Autodesk Fusion 360 part; units mm, degrees
note: some values were not read from the file. Set by a fixed rule: which face or edge a step refers to.
(part 2 of 2)
sketch "Sketch1 (6)" plane through (0, -1, 0) normal (0, -1, 0) x (1, 0, 0) in component "RightBoardHolder"
  circle A0 centre (157, 114) radius 1.35
  circle A1 centre (157, 114) radius 4
  line L0 (157, 118) -> (103, 118)
  line L1 (103, 118) -> (103, 54)
  arc A2 (103, 54) -> (161, 114) centre (100.9655, 114) ccw
  line L2 (103, 118) -> (75, 118)
  line L3 (75, 118) -> (103, 118)
  line L4 (103, 118) -> (103, 54)
  line L5 (103, 54) -> (75, 54)
  line L6 (75, 54) -> (75, 118)
  line L7 (75, 54) -> (95, 54)
  line L8 (95, 54) -> (75, 54)
  line L9 (75, 54) -> (75, 88)
  line L10 (75, 88) -> (95, 88)
  line L11 (95, 88) -> (95, 54)
  dimension "d287" = 54
  dimension "d288" = 64
  dimension "d304" = 28
  dimension "d363" = 20
  dimension "d364" = 34
  constraint coincident A1 L0.start
  constraint horizontal L0
  constraint perpendicular L0 L1
  constraint tangent A1 A2
  constraint coincident A1 A2.end
  constraint perpendicular L1 L2
  constraint horizontal L3
  constraint vertical L4
  constraint horizontal L5
  constraint vertical L6
  constraint perpendicular L6 L7
  constraint horizontal L8
  constraint vertical L9
  constraint horizontal L10
  constraint vertical L11
  measures "d287" distance of L0.start L0.end
  measures "d288" distance of L0.end L1.end
  measures "d304" distance of L0.end L2.end
  measures "d363" distance of L5.end L7.end
  measures "d364" distance of L7.end L10.end
extrude "Extrude1'''''" add sketch "Sketch1 (6)" along normal blind 2 separate body contours A1 | A1 L0 L1 A2 L4 | L1 L2 L3 L4 L5 L6 L10 L11 makes body 8 in component "RightBoardHolder"
sketch "Sketch2 (6)" plane through (0, -1, 0) normal (0, 1, 0) x (-1, 0, 0) in component "RightBoardHolder"
  circle A0 centre (-157, 114) radius 1.35
  arc A1 (-161, 114) -> (-103, 54) centre (-100.9655, 114) ccw
  line L0 (-75, 118) -> (-157, 118)
  arc A2 (-157, 118) -> (-161, 114) centre (-157, 114) ccw
  line L1 (-157, 114) -> (-127, 114)
  line L2 (-127, 114) -> (-95, 114)
  line L3 (-95, 114) -> (-95, 67)
  line L4 (-95, 67) -> (-127, 67)
  line L5 (-127, 67) -> (-127, 114)
  line L6 (-103, 54) -> (-95, 54)
  line L7 (-75, 88) -> (-75, 118)
  line L8 (-95, 88) -> (-75, 88)
  line L9 (-95, 54) -> (-95, 88)
  dimension "d291" = 30
  dimension "d292" = 32
  dimension "d293" = 47
  constraint coincident A0.centre A2.centre
  constraint horizontal L1
  constraint horizontal L2
  constraint vertical L3
  constraint horizontal L4
  constraint vertical L5
  measures "d291" distance of A0.centre L1.end
  measures "d292" distance of L1.end L2.end
  measures "d293" distance of L1.end L4.end
extrude "Extrude2'''''" cut sketch "Sketch2 (6)" against normal blind 1 contours L2 L3 L4 L5 L9 bodies 8 in component "RightBoardHolder"
sketch "Sketch3 (5)" plane through (0, -1, 0) normal (0, 1, 0) x (-1, 0, 0) in component "RightBoardHolder"
  line L0 (-95, 114) -> (-95, 88)
  line L1 (-95, 67) -> (-127, 67)
  line L2 (-127, 67) -> (-127, 114)
  line L3 (-127, 114) -> (-95, 114)
  circle A0 centre (-157, 114) radius 1.35
  arc A1 (-161, 114) -> (-103, 54) centre (-100.9655, 114) ccw
  line L4 (-103, 54) -> (-95, 54)
  line L5 (-75, 88) -> (-75, 118)
  line L6 (-75, 118) -> (-157, 118)
  arc A2 (-157, 118) -> (-161, 114) centre (-157, 114) ccw
  line L7 (-127, 67) -> (-129, 67)
  line L8 (-129, 67) -> (-129, 65)
  line L9 (-129, 65) -> (-127, 65)
  line L10 (-127, 65) -> (-127, 67)
  line L11 (-95, 114) -> (-93, 114)
  line L12 (-93, 114) -> (-93, 116)
  line L13 (-93, 116) -> (-95, 116)
  line L14 (-95, 116) -> (-95, 114)
  line L15 (-93, 116) -> (-129, 116)
  line L16 (-129, 116) -> (-129, 65)
  line L17 (-129, 65) -> (-93, 65)
  line L18 (-93, 65) -> (-93, 116)
  line L19 (-95, 88) -> (-75, 88)
  line L20 (-95, 54) -> (-95, 67)
  line L21 (-111, 65) -> (-111, 67)
  line L22 (-129, 90.5) -> (-127, 90.5)
  dimension "d307" = 2
  dimension "d308" = 2
  dimension "d309" = 2
  dimension "d310" = 2
  constraint horizontal L7
  constraint vertical L8
  constraint horizontal L9
  constraint vertical L10
  constraint coincident L1.end L2.start
  constraint horizontal L11
  constraint vertical L12
  constraint horizontal L13
  constraint vertical L14
  constraint coincident L0.start L3.end
  constraint horizontal L15
  constraint vertical L16
  constraint horizontal L17
  constraint vertical L18
  constraint midpoint L17 L21.start
  constraint midpoint L1 L21.end
  constraint midpoint L16 L22.start
  constraint midpoint L2 L22.end
  measures "d307" distance of L1.end L7.end
  measures "d308" distance of L1.end L9.end
  measures "d309" distance of L0.start L11.end
  measures "d310" distance of L0.start L13.end
extrude "Extrude3'''''" add sketch "Sketch3 (5)" along normal blind 3 contours L11 L12 L13 L14 L15 L18 | L2 L3 L14 L15 L16 L22 | L1 L17 L20 L21 bodies 8 in component "RightBoardHolder"
sketch "Sketch4 (5)" plane through (0, -2, 0) normal (0, 1, 0) x (-1, 0, 0) in component "RightBoardHolder"
  line L0 (-127, 67) -> (-95, 67)
  line L1 (-95, 88) -> (-95, 114)
  line L2 (-95, 114) -> (-127, 114)
  line L3 (-127, 114) -> (-127, 67)
  line L4 (-95, 114) -> (-101, 114)
  line L5 (-101, 114) -> (-101, 111)
  line L6 (-101, 111) -> (-95, 111)
  line L7 (-95, 111) -> (-95, 114)
  circle A0 centre (-101, 111) radius 0.9
  circle A1 centre (-101, 111) radius 2.5
  line L8 (-95, 67) -> (-99, 67)
  line L9 (-99, 67) -> (-99, 71)
  line L10 (-99, 71) -> (-95, 71)
  line L11 (-95, 71) -> (-95, 67)
  circle A2 centre (-99, 71) radius 0.9
  circle A3 centre (-99, 71) radius 2.5
  line L12 (-95, 67) -> (-95, 88)
  dimension "d313" = 6
  dimension "d314" = 3
  dimension "d315" = 1.8
  dimension "d316" = 5
  dimension "d321" = 4
  dimension "d322" = 4
  dimension "d323" = 1.8
  dimension "d324" = 5
  constraint horizontal L4
  constraint vertical L5
  constraint horizontal L6
  constraint vertical L7
  constraint coincident L1.end L2.start
  constraint coincident L5.end L6.start
  constraint concentric A0 A1
  constraint horizontal L8
  constraint vertical L9
  constraint horizontal L10
  constraint vertical L11
  constraint coincident L0.end L8.start
  constraint coincident L9.end L10.start
  constraint concentric A2 A3
  measures "d313" distance of L1.end L4.end
  measures "d314" distance of L1.end L6.end
  measures "d315" diameter of A0
  measures "d316" diameter of A1
  measures "d321" distance of L0.end L8.end
  measures "d322" distance of L0.end L10.end
  measures "d323" diameter of A2
  measures "d324" diameter of A3
extrude "Extrude4'''" cut sketch "Sketch4 (5)" against normal blind 1 contours L9 L10 A2 | L9 L10 A2 | L5 L6 A0 | L5 L6 A0 bodies 8 in component "RightBoardHolder"
extrude "Extrude5'''''" add sketch "Sketch4 (5)" along normal blind 1 contours L9 L10 A2 A3 | L9 L10 A2 A3 | L5 L6 A0 A1 | L5 L6 A0 A1 bodies 8 in component "RightBoardHolder"
sketch "Sketch7 (2)" plane through (0, -1, 0) normal (0, 1, 0) x (-1, 0, 0) in component "RightBoardHolder"
  line L0 (-95, 65) -> (-111, 65)
  line L1 (-129, 90.5) -> (-129, 116)
  line L2 (-129, 116) -> (-93, 116)
  line L3 (-93, 116) -> (-93, 114)
  circle A0 centre (-157, 114) radius 1.35
  line L4 (-95, 88) -> (-75, 88)
  line L5 (-75, 88) -> (-75, 118)
  line L6 (-75, 118) -> (-157, 118)
  arc A1 (-157, 118) -> (-161, 114) centre (-157, 114) ccw
  arc A2 (-161, 114) -> (-103, 54) centre (-100.9655, 114) ccw
  line L7 (-103, 54) -> (-95, 54)
  line L8 (-95, 54) -> (-95, 65)
  line L9 (-75, 88) -> (-75, 98)
  line L10 (-75, 98) -> (-85, 98)
  line L11 (-85, 98) -> (-85, 108)
  line L12 (-85, 108) -> (-75, 108)
  line L13 (-75, 108) -> (-75, 98)
  line L14 (-127, 90.5) -> (-129, 90.5)
  line L15 (-111, 65) -> (-111, 67)
  line L16 (-111, 67) -> (-127, 67)
  line L17 (-127, 67) -> (-127, 90.5)
  line L18 (-93, 114) -> (-95, 114)
  line L19 (-95, 114) -> (-95, 88)
  dimension "d383" = 10
  dimension "d384" = 10
  dimension "d385" = 10
  constraint coincident L4.end L5.start
  constraint perpendicular L4 L9
  constraint horizontal L10
  constraint vertical L11
  constraint horizontal L12
  constraint vertical L13
  measures "d383" distance of L4.end L9.end
  measures "d384" distance of L9.end L10.end
  measures "d385" distance of L9.end L12.end
extrude "Extrude8''" cut sketch "Sketch7 (2)" against normal blind 2 contours L5 L10 L11 L12 L13 bodies 8 in component "RightBoardHolder"
sketch "Sketch10" plane through (0, -1, 0) normal (0, 1, 0) x (-1, 0, 0) in component "LeftBoardHolder"
  line L0 (-69, 91) -> (-69, 118)
  line L1 (-69, 118) -> (-75, 118)
  line L2 (-75, 118) -> (-75, 88)
  line L3 (-75, 88) -> (-55, 88)
  line L4 (-55, 88) -> (-55, 54)
  line L5 (-55, 54) -> (-50.0008, 54)
  arc A0 (-50.0008, 54) -> (-48.9911, 54.1293) centre (-50, 58) ccw
  arc A1 (-48.9911, 54.1293) -> (3.9996, 113.9403) centre (-57.2823, 114.8546) ccw
  arc A2 (3.9996, 113.9403) -> (0, 118) centre (0, 114) ccw
  line L6 (0, 118) -> (-25, 118)
  line L7 (-25, 118) -> (-25, 91)
  line L8 (-25, 91) -> (-69, 91)
  circle A3 centre (0, 114) radius 1.35
  line L9 (-75, 88) -> (-75, 98)
  line L10 (-75, 98) -> (-85, 98)
  line L11 (-85, 98) -> (-85, 108)
  line L12 (-85, 108) -> (-75, 108)
  line L13 (-75, 108) -> (-75, 98)
  dimension "d391" = 10
  dimension "d392" = 10
  dimension "d393" = 10
  constraint coincident L2.end L3.start
  constraint perpendicular L3 L9
  constraint horizontal L10
  constraint vertical L11
  constraint horizontal L12
  constraint vertical L13
  measures "d391" distance of L2.end L9.end
  measures "d392" distance of L9.end L10.end
  measures "d393" distance of L9.end L12.end
extrude "Extrude13" add sketch "Sketch10" against normal blind 2 contours L2 L10 L11 L12 L13 bodies 7 in component "LeftBoardHolder"
sketch "Sketch11" plane through (0, -1, 0) normal (0, 1, 0) x (-1, 0, 0) in component "LeftBoardHolder"
  line L0 (-69, 91) -> (-69, 118)
  line L1 (-69, 118) -> (-75, 118)
  line L2 (-75, 118) -> (-75, 108)
  line L3 (-75, 108) -> (-85, 108)
  line L4 (-85, 108) -> (-85, 98)
  line L5 (-85, 98) -> (-75, 98)
  line L6 (-75, 98) -> (-75, 88)
  line L7 (-75, 88) -> (-55, 88)
  line L8 (-55, 88) -> (-55, 54)
  line L9 (-55, 54) -> (-50.0008, 54)
  arc A0 (-50.0008, 54) -> (-48.9911, 54.1293) centre (-50, 58) ccw
  arc A1 (-48.9911, 54.1293) -> (3.9996, 113.9403) centre (-57.2823, 114.8546) ccw
  arc A2 (3.9996, 113.9403) -> (0, 118) centre (0, 114) ccw
  line L10 (0, 118) -> (-25, 118)
  line L11 (-25, 118) -> (-25, 91)
  line L12 (-25, 91) -> (-69, 91)
  circle A3 centre (0, 114) radius 1.35
  line L13 (-55, 88) -> (-40, 88)
  line L14 (-40, 88) -> (-40, 73)
  line L15 (-40, 73) -> (-55, 73)
  line L16 (-55, 73) -> (-55, 88)
  dimension "d412" = 15
  dimension "d413" = 15
  constraint horizontal L13
  constraint vertical L14
  constraint horizontal L15
  constraint vertical L16
  constraint coincident L7.end L8.start
  measures "d412" distance of L7.end L13.end
  measures "d413" distance of L7.end L15.end
extrude "Extrude14" cut sketch "Sketch11" against normal blind 2 contours L8 L13 L14 L15 L16 | A3 bodies 7 in component "LeftBoardHolder"
fillet "Fillet2''" radius 3 3 edges at (55, -2, 73) (40, -2, 73) (40, -2, 88) on bodies 7 in component "LeftBoardHolder"
fillet "Fillet1''" radius 3 2 edges at (95, -2.5, 88) (95, -2, 54) on bodies 8 in component "RightBoardHolder"
move_face "OffsetFaces4" offset -0.2 5 faces at (75, -2.3333, 114.6667) (81.6667, -2.3333, 108) (75, -2.3333, 94.6667) (85, -2.3333, 101.3333) (78.3333, -2.3333, 98) on bodies 7 in component "LeftBoardHolder"
component "LeftSide" placed x (1, 0, 0) y (0, 1, 0) z (0, 0, 1) at (0, 0, 0)
component "RightSide" placed x (1, 0, 0) y (0, 1, 0) z (0, 0, 1) at (0, 0, 0)
component "LeftBatteryMount" placed x (1, 0, 0) y (0, 1, 0) z (0, 0, 1) at (0, 0, 0) in component "LeftSide"
component "LeftBoardHolder" placed x (1, 0, 0) y (0, 1, 0) z (0, 0, 1) at (0, 0, 0) in component "LeftSide"
component "RightBatteryMount" placed x (1, 0, 0) y (0, 1, 0) z (0, 0, 1) at (0, 0, 0) in component "RightSide"
component "RightBoardHolder" placed x (1, 0, 0) y (0, 1, 0) z (0, 0, 1) at (0, 0, 0) in component "RightSide"
